Autodesk Fusion 360 part; units mm, degrees
(part 8 of 11)
  spline S18 degree 5 poles (-122.968, -126.8819) (-122.9875, -126.9008) (-123.0258, -126.9391) (-123.0815, -126.9984) (-123.1522, -127.0804) (-123.2358, -127.1873) (-123.3161, -127.2972) (-123.3942, -127.4089) (-123.4713, -127.5216) (-123.5476, -127.6349) (-123.623, -127.749) (-123.6973, -127.864) (-123.77, -127.9803) (-123.841, -128.098) (-123.9102, -128.2172) (-123.9778, -128.3376) (-124.0441, -128.459) (-124.1092, -128.5813) (-124.1732, -128.7044) (-124.2363, -128.8282) (-124.2984, -128.9527) (-124.3594, -129.078) (-124.4193, -129.2041) (-124.478, -129.3309) (-124.5356, -129.4586) (-124.5921, -129.5871) (-124.6476, -129.7162) (-124.7021, -129.846) (-124.7556, -129.9764) (-124.8082, -130.1075) (-124.8598, -130.2391) (-124.9105, -130.3714) (-124.9603, -130.5042) (-125.009, -130.6377) (-125.0569, -130.7717) (-125.1038, -130.9063) (-125.1498, -131.0414) (-125.1949, -131.1771) (-125.2391, -131.3133) (-125.2824, -131.45) (-125.3248, -131.5872) (-125.3664, -131.7249) (-125.4071, -131.8631) (-125.4469, -132.0017) (-125.4859, -132.1409) (-125.524, -132.2804) (-125.5613, -132.4205) (-125.5977, -132.561) (-125.6333, -132.7019) (-125.6681, -132.8432) (-125.702, -132.9849) (-125.7351, -133.1271) (-125.7674, -133.2697) (-125.7989, -133.4126) (-125.8295, -133.556) (-125.8594, -133.6997) (-125.8884, -133.8439) (-125.9167, -133.9883) (-125.9441, -134.1332) (-125.9708, -134.2784) (-125.9967, -134.424) (-126.0218, -134.5699) (-126.046, -134.7161) (-126.0696, -134.8627) (-126.0923, -135.0096) (-126.1143, -135.1569) (-126.1354, -135.3044) (-126.1559, -135.4523) (-126.1755, -135.6004) (-126.1944, -135.7489) (-126.2125, -135.8977) (-126.2264, -136.0169) (-126.2365, -136.1065) (-126.243, -136.1663) (-126.2463, -136.1962) knots 0 0 0 0 0 0 0.01428571 0.02857143 0.04285714 0.05714286 0.07142857 0.08571429 0.1 0.11428571 0.12857143 0.14285714 0.15714286 0.17142857 0.18571429 0.2 0.21428571 0.22857143 0.24285714 0.25714286 0.27142857 0.28571429 0.3 0.31428571 0.32857143 0.34285714 0.35714286 0.37142857 0.38571429 0.4 0.41428571 0.42857143 0.44285714 0.45714286 0.47142857 0.48571429 0.5 0.51428571 0.52857143 0.54285714 0.55714286 0.57142857 0.58571429 0.6 0.61428571 0.62857143 0.64285714 0.65714286 0.67142857 0.68571429 0.7 0.71428571 0.72857143 0.74285714 0.75714286 0.77142857 0.78571429 0.8 0.81428571 0.82857143 0.84285714 0.85714286 0.87142857 0.88571429 0.9 0.91428571 0.92857143 0.94285714 0.95714286 0.97142857 0.98571429 1 1 1 1 1 1
  arc A38 (-126.2463, -136.1962) -> (-123.0401, -138.7531) centre (-92.9957, -97.79) ccw
  spline S19 degree 5 poles (-123.0401, -138.7531) (-123.0117, -138.7432) (-122.9548, -138.7235) (-122.8698, -138.6938) (-122.7566, -138.6537) (-122.6156, -138.6029) (-122.475, -138.5515) (-122.3349, -138.4994) (-122.1953, -138.4465) (-122.0562, -138.3931) (-121.9175, -138.3389) (-121.7794, -138.284) (-121.6417, -138.2285) (-121.5045, -138.1723) (-121.3678, -138.1153) (-121.2317, -138.0577) (-121.096, -137.9994) (-120.9609, -137.9404) (-120.8264, -137.8807) (-120.6923, -137.8203) (-120.5588, -137.7593) (-120.4259, -137.6975) (-120.2935, -137.635) (-120.1617, -137.5718) (-120.0305, -137.5078) (-119.8998, -137.4432) (-119.7698, -137.3779) (-119.6403, -137.3118) (-119.5115, -137.2451) (-119.3832, -137.1776) (-119.2556, -137.1093) (-119.1287, -137.0404) (-119.0023, -136.9707) (-118.8767, -136.9003) (-118.7517, -136.8291) (-118.6274, -136.7572) (-118.5037, -136.6845) (-118.3808, -136.6111) (-118.2586, -136.537) (-118.137, -136.4621) (-118.0163, -136.3864) (-117.8962, -136.3099) (-117.777, -136.2327) (-117.6585, -136.1546) (-117.5409, -136.0758) (-117.424, -135.9962) (-117.308, -135.9157) (-117.1927, -135.8345) (-117.0783, -135.7525) (-116.9647, -135.6697) (-116.8521, -135.586) (-116.7404, -135.5014) (-116.6298, -135.4159) (-116.5202, -135.3295) (-116.4117, -135.2422) (-116.3041, -135.1539) (-116.1974, -135.0649) (-116.0917, -134.975) (-115.9869, -134.8844) (-115.8833, -134.7927) (-115.7809, -134.7) (-115.6802, -134.606) (-115.5812, -134.5107) (-115.484, -134.4139) (-115.3884, -134.3159) (-115.294, -134.217) (-115.2004, -134.1174) (-115.1077, -134.0172) (-115.0162, -133.9161) (-114.9269, -133.8134) (-114.8414, -133.7081) (-114.7771, -133.6209) (-114.7318, -133.5535) (-114.7029, -133.5075) (-114.6888, -133.4843) knots -1 -1 -1 -1 -1 -1 -0.98571429 -0.97142857 -0.95714286 -0.94285714 -0.92857143 -0.91428571 -0.9 -0.88571429 -0.87142857 -0.85714286 -0.84285714 -0.82857143 -0.81428571 -0.8 -0.78571429 -0.77142857 -0.75714286 -0.74285714 -0.72857143 -0.71428571 -0.7 -0.68571429 -0.67142857 -0.65714286 -0.64285714 -0.62857143 -0.61428571 -0.6 -0.58571429 -0.57142857 -0.55714286 -0.54285714 -0.52857143 -0.51428571 -0.5 -0.48571429 -0.47142857 -0.45714286 -0.44285714 -0.42857143 -0.41428571 -0.4 -0.38571429 -0.37142857 -0.35714286 -0.34285714 -0.32857143 -0.31428571 -0.3 -0.28571429 -0.27142857 -0.25714286 -0.24285714 -0.22857143 -0.21428571 -0.2 -0.18571429 -0.17142857 -0.15714286 -0.14285714 -0.12857143 -0.11428571 -0.1 -0.08571429 -0.07142857 -0.05714286 -0.04285714 -0.02857143 -0.01428571 0 0 0 0 0 0
  line L19 (-114.6888, -133.4843) -> (-112.5177, -129.913)
  arc A39 (-111.4416, -129.6385) -> (-112.5177, -129.913) centre (-111.8394, -130.3253) ccw
  arc A40 (-111.4416, -129.6385) -> (-106.395, -132.0688) centre (-92.9957, -97.79) ccw
  arc A41 (-105.9388, -133.0812) -> (-106.395, -132.0688) centre (-106.684, -132.808) ccw
  line L20 (-105.9388, -133.0812) -> (-107.3773, -137.0054)
  spline S20 degree 5 poles (-107.3773, -137.0054) (-107.3867, -137.0308) (-107.4046, -137.082) (-107.429, -137.1595) (-107.4571, -137.2642) (-107.4861, -137.3967) (-107.5107, -137.5305) (-107.5327, -137.6651) (-107.5532, -137.8001) (-107.5728, -137.9353) (-107.5912, -138.0708) (-107.6082, -138.2067) (-107.6233, -138.343) (-107.6361, -138.4799) (-107.6468, -138.6172) (-107.6555, -138.755) (-107.6625, -138.8932) (-107.6681, -139.0316) (-107.6724, -139.1703) (-107.6755, -139.3092) (-107.6774, -139.4483) (-107.678, -139.5877) (-107.6773, -139.7272) (-107.6751, -139.867) (-107.6716, -140.0071) (-107.6668, -140.1473) (-107.6608, -140.2877) (-107.6536, -140.4283) (-107.6452, -140.5691) (-107.6357, -140.71) (-107.6251, -140.851) (-107.6134, -140.9921) (-107.6006, -141.1334) (-107.5866, -141.2748) (-107.5716, -141.4163) (-107.5554, -141.5579) (-107.5383, -141.6996) (-107.52, -141.8414) (-107.5007, -141.9833) (-107.4805, -142.1253) (-107.4592, -142.2673) (-107.4369, -142.4094) (-107.4136, -142.5515) (-107.3893, -142.6937) (-107.3641, -142.836) (-107.3378, -142.9783) (-107.3107, -143.1206) (-107.2825, -143.263) (-107.2535, -143.4054) (-107.2235, -143.5478) (-107.1925, -143.6903) (-107.1607, -143.8327) (-107.1279, -143.9752) (-107.0942, -144.1176) (-107.0597, -144.2601) (-107.0242, -144.4026) (-106.9878, -144.545) (-106.9506, -144.6874) (-106.9125, -144.8299) (-106.8735, -144.9723) (-106.8336, -145.1146) (-106.7929, -145.257) (-106.7514, -145.3993) (-106.709, -145.5416) (-106.6657, -145.6838) (-106.6216, -145.826) (-106.5767, -145.9681) (-106.5309, -146.1102) (-106.4843, -146.2522) (-106.4369, -146.3942) (-106.3887, -146.5361) (-106.3495, -146.6495) (-106.3197, -146.7346) (-106.2996, -146.7913) (-106.2896, -146.8197) knots 0 0 0 0 0 0 0.01428571 0.02857143 0.04285714 0.05714286 0.07142857 0.08571429 0.1 0.11428571 0.12857143 0.14285714 0.15714286 0.17142857 0.18571429 0.2 0.21428571 0.22857143 0.24285714 0.25714286 0.27142857 0.28571429 0.3 0.31428571 0.32857143 0.34285714 0.35714286 0.37142857 0.38571429 0.4 0.41428571 0.42857143 0.44285714 0.45714286 0.47142857 0.48571429 0.5 0.51428571 0.52857143 0.54285714 0.55714286 0.57142857 0.58571429 0.6 0.61428571 0.62857143 0.64285714 0.65714286 0.67142857 0.68571429 0.7 0.71428571 0.72857143 0.74285714 0.75714286 0.77142857 0.78571429 0.8 0.81428571 0.82857143 0.84285714 0.85714286 0.87142857 0.88571429 0.9 0.91428571 0.92857143 0.94285714 0.95714286 0.97142857 0.98571429 1 1 1 1 1 1
  arc A42 (-106.2896, -146.8197) -> (-102.2915, -147.7322) centre (-92.9957, -97.79) ccw
  spline S21 degree 5 poles (-102.2915, -147.7322) (-102.2702, -147.711) (-102.2275, -147.6686) (-102.1638, -147.6049) (-102.0792, -147.5197) (-101.9742, -147.4128) (-101.8699, -147.3054) (-101.7663, -147.1977) (-101.6634, -147.0895) (-101.5613, -146.981) (-101.4599, -146.872) (-101.3592, -146.7626) (-101.2592, -146.6528) (-101.16, -146.5426) (-101.0616, -146.4321) (-100.9639, -146.3211) (-100.867, -146.2097) (-100.7709, -146.0979) (-100.6755, -145.9858) (-100.581, -145.8732) (-100.4872, -145.7602) (-100.3942, -145.6469) (-100.3021, -145.5331) (-100.2107, -145.419) (-100.1202, -145.3045) (-100.0306, -145.1896) (-99.9417, -145.0743) (-99.8538, -144.9586) (-99.7666, -144.8425) (-99.6804, -144.7261) (-99.595, -144.6092) (-99.5106, -144.492) (-99.427, -144.3744) (-99.3443, -144.2565) (-99.2626, -144.1381) (-99.1818, -144.0194) (-99.1019, -143.9003) (-99.023, -143.7808) (-98.945, -143.661) (-98.8681, -143.5407) (-98.7921, -143.4202) (-98.7171, -143.2992) (-98.6432, -143.1778) (-98.5703, -143.0561) (-98.4985, -142.9341) (-98.4278, -142.8116) (-98.3581, -142.6888) (-98.2895, -142.5656) (-98.222, -142.4421) (-98.1557, -142.3182) (-98.0905, -142.1939) (-98.0266, -142.0693) (-97.964, -141.9442) (-97.9028, -141.8188) (-97.8428, -141.693) (-97.7842, -141.5669) (-97.7268, -141.4404) (-97.6705, -141.3135) (-97.6154, -141.1864) (-97.5618, -141.0589) (-97.5098, -140.9309) (-97.4598, -140.8025) (-97.412, -140.6737) (-97.3665, -140.5443) (-97.3228, -140.4145) (-97.2807, -140.2844) (-97.2396, -140.1541) (-97.1996, -140.0236) (-97.161, -139.8928) (-97.1251, -139.7616) (-97.0937, -139.6296) (-97.0736, -139.5231) (-97.062, -139.4427) (-97.0559, -139.3888) (-97.0533, -139.3617) knots -1 -1 -1 -1 -1 -1 -0.98571429 -0.97142857 -0.95714286 -0.94285714 -0.92857143 -0.91428571 -0.9 -0.88571429 -0.87142857 -0.85714286 -0.84285714 -0.82857143 -0.81428571 -0.8 -0.78571429 -0.77142857 -0.75714286 -0.74285714 -0.72857143 -0.71428571 -0.7 -0.68571429 -0.67142857 -0.65714286 -0.64285714 -0.62857143 -0.61428571 -0.6 -0.58571429 -0.57142857 -0.55714286 -0.54285714 -0.52857143 -0.51428571 -0.5 -0.48571429 -0.47142857 -0.45714286 -0.44285714 -0.42857143 -0.41428571 -0.4 -0.38571429 -0.37142857 -0.35714286 -0.34285714 -0.32857143 -0.31428571 -0.3 -0.28571429 -0.27142857 -0.25714286 -0.24285714 -0.22857143 -0.21428571 -0.2 -0.18571429 -0.17142857 -0.15714286 -0.14285714 -0.12857143 -0.11428571 -0.1 -0.08571429 -0.07142857 -0.05714286 -0.04285714 -0.02857143 -0.01428571 0 0 0 0 0 0
  line L21 (-97.0533, -139.3617) -> (-96.6467, -135.2021)
  arc A43 (-95.7964, -134.4878) -> (-96.6467, -135.2021) centre (-95.8568, -135.2793) ccw
  arc A44 (-95.7964, -134.4878) -> (-90.1951, -134.4878) centre (-92.9957, -97.79) ccw
  arc A45 (-89.3447, -135.2021) -> (-90.1951, -134.4878) centre (-90.1347, -135.2793) ccw
  line L22 (-89.3447, -135.2021) -> (-88.9382, -139.3617)
  spline S22 degree 5 poles (-88.9382, -139.3617) (-88.9355, -139.3888) (-88.9294, -139.4427) (-88.9178, -139.5231) (-88.8978, -139.6296) (-88.8664, -139.7616) (-88.8305, -139.8928) (-88.7919, -140.0236) (-88.7518, -140.1541) (-88.7108, -140.2844) (-88.6686, -140.4145) (-88.625, -140.5443) (-88.5794, -140.6737) (-88.5316, -140.8025) (-88.4816, -140.9309) (-88.4297, -141.0589) (-88.376, -141.1864) (-88.321, -141.3135) (-88.2647, -141.4404) (-88.2072, -141.5669) (-88.1486, -141.693) (-88.0887, -141.8188) (-88.0274, -141.9442) (-87.9649, -142.0693) (-87.9009, -142.1939) (-87.8358, -142.3182) (-87.7694, -142.4421) (-87.7019, -142.5656) (-87.6333, -142.6888) (-87.5636, -142.8116) (-87.4929, -142.9341) (-87.4211, -143.0561) (-87.3482, -143.1778) (-87.2743, -143.2992) (-87.1994, -143.4202) (-87.1234, -143.5407) (-87.0464, -143.661) (-86.9684, -143.7808) (-86.8895, -143.9003) (-86.8097, -144.0194) (-86.7288, -144.1381) (-86.6471, -144.2565) (-86.5645, -144.3744) (-86.4809, -144.492) (-86.3964, -144.6092) (-86.311, -144.7261) (-86.2248, -144.8425) (-86.1377, -144.9586) (-86.0497, -145.0743) (-85.9609, -145.1896) (-85.8712, -145.3045) (-85.7807, -145.419) (-85.6894, -145.5331) (-85.5972, -145.6469) (-85.5042, -145.7602) (-85.4105, -145.8732) (-85.3159, -145.9858) (-85.2206, -146.0979) (-85.1244, -146.2097) (-85.0275, -146.3211) (-84.9299, -146.4321) (-84.8314, -146.5426) (-84.7322, -146.6528) (-84.6323, -146.7626) (-84.5316, -146.872) (-84.4302, -146.981) (-84.328, -147.0895) (-84.2251, -147.1977) (-84.1215, -147.3054) (-84.0172, -147.4128) (-83.9122, -147.5197) (-83.8276, -147.6049) (-83.7639, -147.6686) (-83.7212, -147.711) (-83.6999, -147.7322) knots 0 0 0 0 0 0 0.01428571 0.02857143 0.04285714 0.05714286 0.07142857 0.08571429 0.1 0.11428571 0.12857143 0.14285714 0.15714286 0.17142857 0.18571429 0.2 0.21428571 0.22857143 0.24285714 0.25714286 0.27142857 0.28571429 0.3 0.31428571 0.32857143 0.34285714 0.35714286 0.37142857 0.38571429 0.4 0.41428571 0.42857143 0.44285714 0.45714286 0.47142857 0.48571429 0.5 0.51428571 0.52857143 0.54285714 0.55714286 0.57142857 0.58571429 0.6 0.61428571 0.62857143 0.64285714 0.65714286 0.67142857 0.68571429 0.7 0.71428571 0.72857143 0.74285714 0.75714286 0.77142857 0.78571429 0.8 0.81428571 0.82857143 0.84285714 0.85714286 0.87142857 0.88571429 0.9 0.91428571 0.92857143 0.94285714 0.95714286 0.97142857 0.98571429 1 1 1 1 1 1
  arc A46 (-83.6999, -147.7322) -> (-79.7018, -146.8197) centre (-92.9957, -97.79) ccw
  spline S23 degree 5 poles (-79.7018, -146.8197) (-79.6918, -146.7913) (-79.6718, -146.7346) (-79.642, -146.6495) (-79.6027, -146.5361) (-79.5545, -146.3942) (-79.5071, -146.2522) (-79.4605, -146.1102) (-79.4148, -145.9681) (-79.3698, -145.826) (-79.3257, -145.6838) (-79.2825, -145.5416) (-79.2401, -145.3993) (-79.1985, -145.257) (-79.1578, -145.1146) (-79.1179, -144.9723) (-79.079, -144.8299) (-79.0408, -144.6874) (-79.0036, -144.545) (-78.9672, -144.4026) (-78.9318, -144.2601) (-78.8972, -144.1176) (-78.8635, -143.9752) (-78.8308, -143.8327) (-78.7989, -143.6903) (-78.768, -143.5478) (-78.738, -143.4054) (-78.7089, -143.263) (-78.6808, -143.1206) (-78.6536, -142.9783) (-78.6274, -142.836) (-78.6021, -142.6937) (-78.5778, -142.5515) (-78.5546, -142.4094) (-78.5323, -142.2673) (-78.511, -142.1253) (-78.4907, -141.9833) (-78.4714, -141.8414) (-78.4532, -141.6996) (-78.436, -141.5579) (-78.4199, -141.4163) (-78.4048, -141.2748) (-78.3908, -141.1334) (-78.378, -140.9921) (-78.3663, -140.851) (-78.3557, -140.71) (-78.3462, -140.5691) (-78.3379, -140.4283) (-78.3306, -140.2877) (-78.3246, -140.1473) (-78.3198, -140.0071) (-78.3163, -139.867) (-78.3142, -139.7272) (-78.3134, -139.5877) (-78.314, -139.4483) (-78.3159, -139.3092) (-78.319, -139.1703) (-78.3234, -139.0316) (-78.3289, -138.8932) (-78.3359, -138.755) (-78.3446, -138.6172) (-78.3553, -138.4799) (-78.3681, -138.343) (-78.3832, -138.2067) (-78.4002, -138.0708) (-78.4187, -137.9353) (-78.4382, -137.8001) (-78.4588, -137.6651) (-78.4807, -137.5305) (-78.5053, -137.3967) (-78.5343, -137.2642) (-78.5624, -137.1595) (-78.5869, -137.082) (-78.6048, -137.0308) (-78.6141, -137.0054) knots -1 -1 -1 -1 -1 -1 -0.98571429 -0.97142857 -0.95714286 -0.94285714 -0.92857143 -0.91428571 -0.9 -0.88571429 -0.87142857 -0.85714286 -0.84285714 -0.82857143 -0.81428571 -0.8 -0.78571429 -0.77142857 -0.75714286 -0.74285714 -0.72857143 -0.71428571 -0.7 -0.68571429 -0.67142857 -0.65714286 -0.64285714 -0.62857143 -0.61428571 -0.6 -0.58571429 -0.57142857 -0.55714286 -0.54285714 -0.52857143 -0.51428571 -0.5 -0.48571429 -0.47142857 -0.45714286 -0.44285714 -0.42857143 -0.41428571 -0.4 -0.38571429 -0.37142857 -0.35714286 -0.34285714 -0.32857143 -0.31428571 -0.3 -0.28571429 -0.27142857 -0.25714286 -0.24285714 -0.22857143 -0.21428571 -0.2 -0.18571429 -0.17142857 -0.15714286 -0.14285714 -0.12857143 -0.11428571 -0.1 -0.08571429 -0.07142857 -0.05714286 -0.04285714 -0.02857143 -0.01428571 0 0 0 0 0 0
  line L23 (-78.6141, -137.0054) -> (-80.0527, -133.0812)
  arc A47 (-79.5964, -132.0688) -> (-80.0527, -133.0812) centre (-79.3074, -132.808) ccw
  arc A48 (-79.5964, -132.0688) -> (-74.5498, -129.6385) centre (-92.9957, -97.79) ccw
  arc A49 (-73.4737, -129.913) -> (-74.5498, -129.6385) centre (-74.152, -130.3253) ccw
  line L24 (-73.4737, -129.913) -> (-71.3027, -133.4843)
  spline S24 degree 5 poles (-71.3027, -133.4843) (-71.2886, -133.5075) (-71.2597, -133.5535) (-71.2143, -133.6209) (-71.1501, -133.7081) (-71.0645, -133.8134) (-70.9752, -133.9161) (-70.8837, -134.0172) (-70.791, -134.1174) (-70.6974, -134.217) (-70.603, -134.3159) (-70.5074, -134.4139) (-70.4102, -134.5107) (-70.3112, -134.606) (-70.2105, -134.7) (-70.1082, -134.7927) (-70.0045, -134.8844) (-69.8997, -134.975) (-69.794, -135.0649) (-69.6874, -135.1539) (-69.5798, -135.2422) (-69.4712, -135.3295) (-69.3616, -135.4159) (-69.251, -135.5014) (-69.1393, -135.586) (-69.0267, -135.6697) (-68.9131, -135.7525) (-68.7987, -135.8345) (-68.6835, -135.9157) (-68.5674, -135.9962) (-68.4506, -136.0758) (-68.3329, -136.1546) (-68.2145, -136.2327) (-68.0952, -136.3099) (-67.9752, -136.3864) (-67.8544, -136.4621) (-67.7329, -136.537) (-67.6106, -136.6111) (-67.4877, -136.6845) (-67.3641, -136.7572) (-67.2398, -136.8291) (-67.1148, -136.9003) (-66.9891, -136.9707) (-66.8628, -137.0404) (-66.7358, -137.1093) (-66.6082, -137.1776) (-66.48, -137.2451) (-66.3511, -137.3118) (-66.2217, -137.3779) (-66.0916, -137.4432) (-65.961, -137.5078) (-65.8297, -137.5718) (-65.6979, -137.635) (-65.5656, -137.6975) (-65.4326, -137.7593) (-65.2991, -137.8203) (-65.1651, -137.8807) (-65.0305, -137.9404) (-64.8954, -137.9994) (-64.7598, -138.0577) (-64.6236, -138.1153) (-64.4869, -138.1723) (-64.3498, -138.2285) (-64.2121, -138.284) (-64.0739, -138.3389) (-63.9352, -138.3931) (-63.7961, -138.4465) (-63.6565, -138.4994) (-63.5164, -138.5515) (-63.3759, -138.6029) (-63.2349, -138.6537) (-63.1217, -138.6938) (-63.0366, -138.7235) (-62.9798, -138.7432) (-62.9513, -138.7531) knots 0 0 0 0 0 0 0.01428571 0.02857143 0.04285714 0.05714286 0.07142857 0.08571429 0.1 0.11428571 0.12857143 0.14285714 0.15714286 0.17142857 0.18571429 0.2 0.21428571 0.22857143 0.24285714 0.25714286 0.27142857 0.28571429 0.3 0.31428571 0.32857143 0.34285714 0.35714286 0.37142857 0.38571429 0.4 0.41428571 0.42857143 0.44285714 0.45714286 0.47142857 0.48571429 0.5 0.51428571 0.52857143 0.54285714 0.55714286 0.57142857 0.58571429 0.6 0.61428571 0.62857143 0.64285714 0.65714286 0.67142857 0.68571429 0.7 0.71428571 0.72857143 0.74285714 0.75714286 0.77142857 0.78571429 0.8 0.81428571 0.82857143 0.84285714 0.85714286 0.87142857 0.88571429 0.9 0.91428571 0.92857143 0.94285714 0.95714286 0.97142857 0.98571429 1 1 1 1 1 1
  arc A50 (-62.9513, -138.7531) -> (-59.7452, -136.1962) centre (-92.9957, -97.79) ccw
  spline S25 degree 5 poles (-59.7452, -136.1962) (-59.7484, -136.1663) (-59.755, -136.1065) (-59.765, -136.0169) (-59.7789, -135.8977) (-59.797, -135.7489) (-59.8159, -135.6004) (-59.8356, -135.4523) (-59.856, -135.3044) (-59.8772, -135.1569) (-59.8991, -135.0096) (-59.9219, -134.8627) (-59.9454, -134.7161) (-59.9697, -134.5699) (-59.9948, -134.424) (-60.0206, -134.2784) (-60.0473, -134.1332) (-60.0747, -133.9883) (-60.103, -133.8439) (-60.132, -133.6997) (-60.1619, -133.556) (-60.1926, -133.4126) (-60.224, -133.2697) (-60.2563, -133.1271) (-60.2894, -132.9849) (-60.3234, -132.8432) (-60.3581, -132.7019) (-60.3937, -132.561) (-60.4302, -132.4205) (-60.4674, -132.2804) (-60.5055, -132.1409) (-60.5445, -132.0017) (-60.5843, -131.8631) (-60.625, -131.7249) (-60.6666, -131.5872) (-60.709, -131.45) (-60.7524, -131.3133) (-60.7966, -131.1771) (-60.8417, -131.0414) (-60.8877, -130.9063) (-60.9346, -130.7717) (-60.9824, -130.6377) (-61.0312, -130.5042) (-61.0809, -130.3714) (-61.1316, -130.2391) (-61.1832, -130.1075) (-61.2358, -129.9764) (-61.2893, -129.846) (-61.3438, -129.7162) (-61.3993, -129.5871) (-61.4558, -129.4586) (-61.5135, -129.3309) (-61.5722, -129.2041) (-61.6321, -129.078) (-61.6931, -128.9527) (-61.7551, -128.8282) (-61.8182, -128.7044) (-61.8823, -128.5813) (-61.9474, -128.459) (-62.0136, -128.3376) (-62.0812, -128.2172) (-62.1505, -128.098) (-62.2214, -127.9803) (-62.2941, -127.864) (-62.3684, -127.749) (-62.4438, -127.6349) (-62.5201, -127.5216) (-62.5972, -127.4089) (-62.6754, -127.2972) (-62.7556, -127.1873) (-62.8392, -127.0804) (-62.9099, -126.9984) (-62.9656, -126.9391) (-63.0039, -126.9008) (-63.0234, -126.8819) knots -1 -1 -1 -1 -1 -1 -0.98571429 -0.97142857 -0.95714286 -0.94285714 -0.92857143 -0.91428571 -0.9 -0.88571429 -0.87142857 -0.85714286 -0.84285714 -0.82857143 -0.81428571 -0.8 -0.78571429 -0.77142857 -0.75714286 -0.74285714 -0.72857143 -0.71428571 -0.7 -0.68571429 -0.67142857 -0.65714286 -0.64285714 -0.62857143 -0.61428571 -0.6 -0.58571429 -0.57142857 -0.55714286 -0.54285714 -0.52857143 -0.51428571 -0.5 -0.48571429 -0.47142857 -0.45714286 -0.44285714 -0.42857143 -0.41428571 -0.4 -0.38571429 -0.37142857 -0.35714286 -0.34285714 -0.32857143 -0.31428571 -0.3 -0.28571429 -0.27142857 -0.25714286 -0.24285714 -0.22857143 -0.21428571 -0.2 -0.18571429 -0.17142857 -0.15714286 -0.14285714 -0.12857143 -0.11428571 -0.1 -0.08571429 -0.07142857 -0.05714286 -0.04285714 -0.02857143 -0.01428571 0 0 0 0 0 0
  line L25 (-63.0234, -126.8819) -> (-66.0221, -123.9705)
  arc A51 (-66.0503, -122.8603) -> (-66.0221, -123.9705) centre (-65.4692, -123.401) ccw
  arc A52 (-66.0503, -122.8603) -> (-62.558, -118.4811) centre (-92.9957, -97.79) ccw
  arc A53 (-61.4694, -118.2616) -> (-62.558, -118.4811) centre (-61.9015, -118.9273) ccw
  line L26 (-61.4694, -118.2616) -> (-57.9637, -120.5372)
  spline S26 degree 5 poles (-57.9637, -120.5372) (-57.941, -120.552) (-57.895, -120.5808) (-57.8249, -120.6219) (-57.7292, -120.6726) (-57.6064, -120.7304) (-57.4814, -120.7841) (-57.3551, -120.8355) (-57.2281, -120.8856) (-57.1006, -120.9347) (-56.9726, -120.9829) (-56.8439, -121.0297) (-56.7144, -121.0747) (-56.5838, -121.1177) (-56.4523, -121.1587) (-56.3198, -121.1978) (-56.1867, -121.2354) (-56.053, -121.2716) (-55.9187, -121.3067) (-55.784, -121.3406) (-55.6488, -121.3734) (-55.5131, -121.405) (-55.3768, -121.4353) (-55.2401, -121.4644) (-55.1028, -121.4921) (-54.965, -121.5186) (-54.8267, -121.544) (-54.6881, -121.5682) (-54.549, -121.5914) (-54.4095, -121.6135) (-54.2697, -121.6346) (-54.1295, -121.6546) (-53.9889, -121.6735) (-53.8479, -121.6913) (-53.7066, -121.7081) (-53.565, -121.7239) (-53.423, -121.7387) (-53.2807, -121.7525) (-53.1381, -121.7653) (-52.9951, -121.7771) (-52.8519, -121.7879) (-52.7085, -121.7978) (-52.5647, -121.8067) (-52.4206, -121.8147) (-52.2763, -121.8217) (-52.1318, -121.8278) (-51.9869, -121.833) (-51.8419, -121.8373) (-51.6966, -121.8406) (-51.5511, -121.8431) (-51.4053, -121.8446) (-51.2593, -121.8452) (-51.1132, -121.845) (-50.9668, -121.8439) (-50.8202, -121.8419) (-50.6734, -121.839) (-50.5264, -121.8352) (-50.3793, -121.8306) (-50.232, -121.8252) (-50.0845, -121.8188) (-49.9368, -121.8117) (-49.789, -121.8037) (-49.641, -121.7948) (-49.4928, -121.7851) (-49.3445, -121.7746) (-49.1961, -121.7632) (-49.0475, -121.751) (-48.8988, -121.738) (-48.75, -121.7242) (-48.6011, -121.7096) (-48.452, -121.6942) (-48.3326, -121.6812) (-48.2431, -121.6711) (-48.1833, -121.6642) (-48.1534, -121.6607) knots 0 0 0 0 0 0 0.01428571 0.02857143 0.04285714 0.05714286 0.07142857 0.08571429 0.1 0.11428571 0.12857143 0.14285714 0.15714286 0.17142857 0.18571429 0.2 0.21428571 0.22857143 0.24285714 0.25714286 0.27142857 0.28571429 0.3 0.31428571 0.32857143 0.34285714 0.35714286 0.37142857 0.38571429 0.4 0.41428571 0.42857143 0.44285714 0.45714286 0.47142857 0.48571429 0.5 0.51428571 0.52857143 0.54285714 0.55714286 0.57142857 0.58571429 0.6 0.61428571 0.62857143 0.64285714 0.65714286 0.67142857 0.68571429 0.7 0.71428571 0.72857143 0.74285714 0.75714286 0.77142857 0.78571429 0.8 0.81428571 0.82857143 0.84285714 0.85714286 0.87142857 0.88571429 0.9 0.91428571 0.92857143 0.94285714 0.95714286 0.97142857 0.98571429 1 1 1 1 1 1
  arc A54 (-48.1534, -121.6607) -> (-46.3741, -117.9659) centre (-92.9957, -97.79) ccw
  spline S27 degree 5 poles (-46.3741, -117.9659) (-46.39, -117.9404) (-46.4219, -117.8894) (-46.4698, -117.813) (-46.5341, -117.7116) (-46.615, -117.5854) (-46.6964, -117.4599) (-46.7784, -117.3349) (-46.8609, -117.2105) (-46.9441, -117.0868) (-47.0277, -116.9637) (-47.112, -116.8412) (-47.1967, -116.7193) (-47.2821, -116.5981) (-47.368, -116.4775) (-47.4545, -116.3576) (-47.5415, -116.2383) (-47.6291, -116.1197) (-47.7172, -116.0018) (-47.8059, -115.8845) (-47.8952, -115.768) (-47.985, -115.6521) (-48.0754, -115.537) (-48.1663, -115.4225) (-48.2578, -115.3088) (-48.3499, -115.1958) (-48.4426, -115.0836) (-48.5358, -114.9721) (-48.6295, -114.8613) (-48.7239, -114.7513) (-48.8188, -114.6421) (-48.9143, -114.5336) (-49.0103, -114.426) (-49.1069, -114.3192) (-49.2041, -114.2131) (-49.3019, -114.1079) (-49.4002, -114.0036) (-49.4991, -113.9) (-49.5986, -113.7974) (-49.6987, -113.6956) (-49.7994, -113.5947) (-49.9006, -113.4947) (-50.0025, -113.3956) (-50.1049, -113.2975) (-50.208, -113.2003) (-50.3116, -113.1041) (-50.4158, -113.0089) (-50.5207, -112.9146) (-50.6261, -112.8213) (-50.7321, -112.729) (-50.8388, -112.6378) (-50.9461, -112.5478) (-51.054, -112.4589) (-51.1627, -112.3713) (-51.272, -112.2849) (-51.3819, -112.1997) (-51.4925, -112.1155) (-51.6036, -112.0324) (-51.7153, -111.9504) (-51.8277, -111.8698) (-51.9409, -111.7906) (-52.0549, -111.7133) (-52.1699, -111.6381) (-52.2859, -111.5649) (-52.4027, -111.4934) (-52.5202, -111.4234) (-52.6381, -111.3544) (-52.7564, -111.2863) (-52.8753, -111.2195) (-52.9953, -111.1553) (-53.117, -111.0954) (-53.2163, -111.0521) (-53.2922, -111.0229) (-53.3434, -111.005) (-53.3691, -110.9964) knots -1 -1 -1 -1 -1 -1 -0.98571429 -0.97142857 -0.95714286 -0.94285714 -0.92857143 -0.91428571 -0.9 -0.88571429 -0.87142857 -0.85714286 -0.84285714 -0.82857143 -0.81428571 -0.8 -0.78571429 -0.77142857 -0.75714286 -0.74285714 -0.72857143 -0.71428571 -0.7 -0.68571429 -0.67142857 -0.65714286 -0.64285714 -0.62857143 -0.61428571 -0.6 -0.58571429 -0.57142857 -0.55714286 -0.54285714 -0.52857143 -0.51428571 -0.5 -0.48571429 -0.47142857 -0.45714286 -0.44285714 -0.42857143 -0.41428571 -0.4 -0.38571429 -0.37142857 -0.35714286 -0.34285714 -0.32857143 -0.31428571 -0.3 -0.28571429 -0.27142857 -0.25714286 -0.24285714 -0.22857143 -0.21428571 -0.2 -0.18571429 -0.17142857 -0.15714286 -0.14285714 -0.12857143 -0.11428571 -0.1 -0.08571429 -0.07142857 -0.05714286 -0.04285714 -0.02857143 -0.01428571 0 0 0 0 0 0
  line L27 (-53.3691, -110.9964) -> (-57.334, -109.6744)
  arc A55 (-57.8411, -108.6864) -> (-57.334, -109.6744) centre (-57.083, -108.9214) ccw
  circle A56 centre (-92.9957, -97.79) radius 5
  circle A57 centre (-92.9957, -97.79) radius 10 construction
  line L28 (-102.9957, -87.79) -> (-82.9957, -87.79)
  line L29 (-82.9957, -87.79) -> (-82.9957, -107.79)
  line L30 (-82.9957, -107.79) -> (-102.9957, -107.79)
  line L31 (-102.9957, -107.79) -> (-102.9957, -87.79)
  dimension "d112" = 5
  dimension "d113" = 20
  dimension "d114" = 20
  constraint horizontal L28
  constraint vertical L29
  constraint horizontal L30
  constraint vertical L31
  constraint tangent A57 L28
  constraint tangent A57 L29
  measures "d112" distance of A56
  measures "d113" distance of L28.start L28.end
  measures "d114" distance of L28.end L29.end
extrude "Extrude3'" add sketch "Sketch4" along normal blind 20 contours L28 L29 L30 L31 sketch seen with x (1, 0, 0) y (0, 1, 0) z (0, 0, 1) at (12.0054, 91.2413, 0) bodies 2 in component "Spur Gear (14 teeth)"
sketch "Sketch5" plane through (0, 0, 12.5) normal (0, 0, -1) x (-1, 0, 0)
  circle A0 centre (-50, -10) radius 2.75
  circle A1 centre (50, 10) radius 2.75
  circle A2 centre (-50, 10) radius 2.75
  circle A3 centre (50, -10) radius 2.75
  circle A4 centre (0.5538, 0.6546) radius 15.5
  arc A5 (-75.7049, -29.609) -> (-75.2572, -28.5856) centre (-75.9978, -28.8713) ccw
  line L0 (-75.7049, -29.609) -> (-77.0937, -30.1604)
  spline S0 degree 5 poles (-77.0937, -30.1604) (-77.1259, -30.1732) (-77.1899, -30.1995) (-77.2849, -30.2412) (-77.4095, -30.3012) (-77.5625, -30.3821) (-77.7135, -30.4672) (-77.8634, -30.5549) (-78.0125, -30.644) (-78.1613, -30.7341) (-78.3095, -30.8251) (-78.4571, -30.9174) (-78.6037, -31.0115) (-78.7494, -31.1075) (-78.894, -31.2056) (-79.0377, -31.3055) (-79.1805, -31.407) (-79.3226, -31.5098) (-79.4641, -31.6138) (-79.605, -31.7187) (-79.7453, -31.8248) (-79.885, -31.9319) (-80.024, -32.0402) (-80.1623, -32.1498) (-80.2999, -32.2605) (-80.4368, -32.3724) (-80.5731, -32.4853) (-80.7088, -32.5993) (-80.8439, -32.7142) (-80.9784, -32.8301) (-81.1124, -32.9469) (-81.2457, -33.0647) (-81.3785, -33.1834) (-81.5106, -33.303) (-81.6422, -33.4236) (-81.7732, -33.545) (-81.9037, -33.6674) (-82.0336, -33.7906) (-82.1629, -33.9146) (-82.2917, -34.0395) (-82.4199, -34.1651) (-82.5476, -34.2916) (-82.6747, -34.4189) (-82.8013, -34.547) (-82.9273, -34.6759) (-83.0528, -34.8055) (-83.1778, -34.936) (-83.3022, -35.0671) (-83.4261, -35.199) (-83.5495, -35.3317) (-83.6723, -35.4651) (-83.7947, -35.5992) (-83.9165, -35.734) (-84.0377, -35.8695) (-84.1585, -36.0057) (-84.2787, -36.1426) (-84.3985, -36.2802) (-84.5177, -36.4185) (-84.6364, -36.5574) (-84.7546, -36.697) (-84.8723, -36.8372) (-84.9894, -36.9781) (-85.1061, -37.1197) (-85.2222, -37.2619) (-85.3379, -37.4047) (-85.453, -37.5482) (-85.5677, -37.6922) (-85.6818, -37.8369) (-85.7955, -37.9822) (-85.9086, -38.1281) (-86.0212, -38.2746) (-86.111, -38.3923) (-86.178, -38.4808) (-86.2226, -38.54) (-86.2449, -38.5696) knots 0 0 0 0 0 0 0.01428571 0.02857143 0.04285714 0.05714286 0.07142857 0.08571429 0.1 0.11428571 0.12857143 0.14285714 0.15714286 0.17142857 0.18571429 0.2 0.21428571 0.22857143 0.24285714 0.25714286 0.27142857 0.28571429 0.3 0.31428571 0.32857143 0.34285714 0.35714286 0.37142857 0.38571429 0.4 0.41428571 0.42857143 0.44285714 0.45714286 0.47142857 0.48571429 0.5 0.51428571 0.52857143 0.54285714 0.55714286 0.57142857 0.58571429 0.6 0.61428571 0.62857143 0.64285714 0.65714286 0.67142857 0.68571429 0.7 0.71428571 0.72857143 0.74285714 0.75714286 0.77142857 0.78571429 0.8 0.81428571 0.82857143 0.84285714 0.85714286 0.87142857 0.88571429 0.9 0.91428571 0.92857143 0.94285714 0.95714286 0.97142857 0.98571429 1 1 1 1 1 1
  arc A6 (-86.2449, -38.5696) -> (-84.231, -42.7515) centre (0.5538, 0.6546) ccw
  spline S1 degree 5 poles (-71.9508, -40.8398) (-71.9808, -40.857) (-72.0413, -40.8906) (-72.1332, -40.9389) (-72.2578, -40.9989) (-72.4164, -41.0681) (-72.5771, -41.1331) (-72.7391, -41.1956) (-72.9018, -41.2566) (-73.0649, -41.3168) (-73.2285, -41.3759) (-73.3927, -41.4337) (-73.5577, -41.4898) (-73.7236, -41.5437) (-73.8904, -41.5957) (-74.0581, -41.6457) (-74.2265, -41.6941) (-74.3955, -41.7411) (-74.565, -41.7869) (-74.7349, -41.8316) (-74.9053, -41.8752) (-75.0761, -41.9176) (-75.2475, -41.9587) (-75.4193, -41.9985) (-75.5917, -42.0371) (-75.7646, -42.0744) (-75.9378, -42.1105) (-76.1116, -42.1456) (-76.2856, -42.1795) (-76.4601, -42.2125) (-76.635, -42.2443) (-76.8102, -42.2752) (-76.9858, -42.305) (-77.1617, -42.3337) (-77.338, -42.3614) (-77.5146, -42.3881) (-77.6916, -42.4138) (-77.8689, -42.4386) (-78.0465, -42.4623) (-78.2244, -42.4852) (-78.4026, -42.5071) (-78.5811, -42.528) (-78.7599, -42.548) (-78.939, -42.5671) (-79.1183, -42.5853) (-79.2979, -42.6026) (-79.4778, -42.619) (-79.658, -42.6345) (-79.8383, -42.6491) (-80.019, -42.6629) (-80.1998, -42.6758) (-80.381, -42.6878) (-80.5623, -42.699) (-80.7439, -42.7093) (-80.9257, -42.7188) (-81.1077, -42.7274) (-81.2899, -42.7353) (-81.4723, -42.7423) (-81.6549, -42.7484) (-81.8378, -42.7538) (-82.0208, -42.7584) (-82.204, -42.7621) (-82.3874, -42.7651) (-82.571, -42.7672) (-82.7548, -42.7686) (-82.9387, -42.7692) (-83.1228, -42.769) (-83.3071, -42.768) (-83.4916, -42.7663) (-83.6762, -42.7638) (-83.861, -42.7605) (-84.0089, -42.7573) (-84.1199, -42.7545) (-84.194, -42.7525) (-84.231, -42.7515) knots 0 0 0 0 0 0 0.01428571 0.02857143 0.04285714 0.05714286 0.07142857 0.08571429 0.1 0.11428571 0.12857143 0.14285714 0.15714286 0.17142857 0.18571429 0.2 0.21428571 0.22857143 0.24285714 0.25714286 0.27142857 0.28571429 0.3 0.31428571 0.32857143 0.34285714 0.35714286 0.37142857 0.38571429 0.4 0.41428571 0.42857143 0.44285714 0.45714286 0.47142857 0.48571429 0.5 0.51428571 0.52857143 0.54285714 0.55714286 0.57142857 0.58571429 0.6 0.61428571 0.62857143 0.64285714 0.65714286 0.67142857 0.68571429 0.7 0.71428571 0.72857143 0.74285714 0.75714286 0.77142857 0.78571429 0.8 0.81428571 0.82857143 0.84285714 0.85714286 0.87142857 0.88571429 0.9 0.91428571 0.92857143 0.94285714 0.95714286 0.97142857 0.98571429 1 1 1 1 1 1
  line L1 (-71.9508, -40.8398) -> (-70.6538, -40.0978)
  arc A7 (-69.5745, -40.3858) -> (-70.6538, -40.0978) centre (-70.2596, -40.7867) ccw
  arc A8 (-69.5745, -40.3858) -> (-66.8499, -44.7221) centre (0.5538, 0.6546) ccw
  arc A9 (-67.0586, -45.8194) -> (-66.8499, -44.7221) centre (-67.5084, -45.1653) ccw
  line L2 (-67.0586, -45.8194) -> (-68.2899, -46.666)
  spline S2 degree 5 poles (-68.2899, -46.666) (-68.3185, -46.6856) (-68.375, -46.7255) (-68.4583, -46.7874) (-68.5664, -46.8736) (-68.6976, -46.9865) (-68.826, -47.103) (-68.9525, -47.2219) (-69.0781, -47.342) (-69.2031, -47.4628) (-69.3273, -47.5846) (-69.4506, -47.7074) (-69.5727, -47.8317) (-69.6933, -47.9578) (-69.8125, -48.0856) (-69.9303, -48.215) (-70.047, -48.3457) (-70.1627, -48.4776) (-70.2775, -48.6104) (-70.3915, -48.7441) (-70.5047, -48.8787) (-70.617, -49.0142) (-70.7284, -49.1508) (-70.8389, -49.2883) (-70.9484, -49.4269) (-71.057, -49.5664) (-71.1647, -49.7069) (-71.2717, -49.8482) (-71.3778, -49.9903) (-71.4832, -50.1332) (-71.5878, -50.2769) (-71.6916, -50.4214) (-71.7946, -50.5667) (-71.8968, -50.7127) (-71.9983, -50.8595) (-72.099, -51.0071) (-72.1989, -51.1554) (-72.2982, -51.3044) (-72.3966, -51.4541) (-72.4944, -51.6045) (-72.5914, -51.7555) (-72.6878, -51.9073) (-72.7834, -52.0596) (-72.8783, -52.2127) (-72.9725, -52.3664) (-73.066, -52.5207) (-73.1588, -52.6757) (-73.2509, -52.8312) (-73.3424, -52.9874) (-73.4331, -53.1442) (-73.5232, -53.3016) (-73.6126, -53.4595) (-73.7014, -53.618) (-73.7895, -53.7772) (-73.8769, -53.9368) (-73.9637, -54.097) (-74.0498, -54.2578) (-74.1352, -54.4191) (-74.22, -54.581) (-74.3042, -54.7434) (-74.3877, -54.9063) (-74.4706, -55.0698) (-74.5528, -55.2337) (-74.6344, -55.3982) (-74.7154, -55.5632) (-74.7958, -55.7287) (-74.8755, -55.8946) (-74.9545, -56.0611) (-75.033, -56.228) (-75.1108, -56.3954) (-75.1881, -56.5633) (-75.2493, -56.698) (-75.295, -56.7993) (-75.3253, -56.8669) (-75.3405, -56.9007) knots 0 0 0 0 0 0 0.01428571 0.02857143 0.04285714 0.05714286 0.07142857 0.08571429 0.1 0.11428571 0.12857143 0.14285714 0.15714286 0.17142857 0.18571429 0.2 0.21428571 0.22857143 0.24285714 0.25714286 0.27142857 0.28571429 0.3 0.31428571 0.32857143 0.34285714 0.35714286 0.37142857 0.38571429 0.4 0.41428571 0.42857143 0.44285714 0.45714286 0.47142857 0.48571429 0.5 0.51428571 0.52857143 0.54285714 0.55714286 0.57142857 0.58571429 0.6 0.61428571 0.62857143 0.64285714 0.65714286 0.67142857 0.68571429 0.7 0.71428571 0.72857143 0.74285714 0.75714286 0.77142857 0.78571429 0.8 0.81428571 0.82857143 0.84285714 0.85714286 0.87142857 0.88571429 0.9 0.91428571 0.92857143 0.94285714 0.95714286 0.97142857 0.98571429 1 1 1 1 1 1
  arc A10 (-75.3405, -56.9007) -> (-72.4465, -60.5296) centre (0.5538, 0.6546) ccw
  spline S3 degree 5 poles (-60.8996, -55.9332) (-60.925, -55.9567) (-60.9765, -56.003) (-61.0553, -56.0704) (-61.1634, -56.1566) (-61.3027, -56.2594) (-61.4449, -56.3586) (-61.5889, -56.4555) (-61.7339, -56.5513) (-61.8796, -56.6462) (-62.0259, -56.7402) (-62.1731, -56.8331) (-62.3215, -56.9245) (-62.4713, -57.014) (-62.6224, -57.1018) (-62.7747, -57.1878) (-62.9282, -57.2725) (-63.0824, -57.3559) (-63.2375, -57.4383) (-63.3932, -57.5197) (-63.5496, -57.6001) (-63.7067, -57.6795) (-63.8646, -57.7577) (-64.0233, -57.8347) (-64.1828, -57.9107) (-64.343, -57.9855) (-64.5039, -58.0593) (-64.6655, -58.1321) (-64.8276, -58.204) (-64.9904, -58.2749) (-65.1538, -58.3449) (-65.3177, -58.4139) (-65.4823, -58.4821) (-65.6474, -58.5492) (-65.8131, -58.6155) (-65.9794, -58.6808) (-66.1462, -58.7453) (-66.3135, -58.8088) (-66.4814, -58.8715) (-66.6498, -58.9334) (-66.8186, -58.9944) (-66.988, -59.0545) (-67.1579, -59.1138) (-67.3282, -59.1723) (-67.499, -59.2299) (-67.6703, -59.2868) (-67.842, -59.3428) (-68.0141, -59.398) (-68.1868, -59.4524) (-68.3598, -59.506) (-68.5333, -59.5588) (-68.7072, -59.6108) (-68.8815, -59.662) (-69.0562, -59.7125) (-69.2313, -59.7622) (-69.4068, -59.8112) (-69.5827, -59.8593) (-69.759, -59.9067) (-69.9357, -59.9534) (-70.1127, -59.9993) (-70.2902, -60.0445) (-70.468, -60.0889) (-70.6461, -60.1326) (-70.8246, -60.1756) (-71.0035, -60.2178) (-71.1827, -60.2593) (-71.3622, -60.3001) (-71.5421, -60.3402) (-71.7223, -60.3795) (-71.9029, -60.4181) (-72.0837, -60.4561) (-72.2287, -60.4858) (-72.3375, -60.5078) (-72.4102, -60.5224) (-72.4465, -60.5296) knots 0 0 0 0 0 0 0.01428571 0.02857143 0.04285714 0.05714286 0.07142857 0.08571429 0.1 0.11428571 0.12857143 0.14285714 0.15714286 0.17142857 0.18571429 0.2 0.21428571 0.22857143 0.24285714 0.25714286 0.27142857 0.28571429 0.3 0.31428571 0.32857143 0.34285714 0.35714286 0.37142857 0.38571429 0.4 0.41428571 0.42857143 0.44285714 0.45714286 0.47142857 0.48571429 0.5 0.51428571 0.52857143 0.54285714 0.55714286 0.57142857 0.58571429 0.6 0.61428571 0.62857143 0.64285714 0.65714286 0.67142857 0.68571429 0.7 0.71428571 0.72857143 0.74285714 0.75714286 0.77142857 0.78571429 0.8 0.81428571 0.82857143 0.84285714 0.85714286 0.87142857 0.88571429 0.9 0.91428571 0.92857143 0.94285714 0.95714286 0.97142857 0.98571429 1 1 1 1 1 1
  line L3 (-60.8996, -55.9332) -> (-59.8002, -54.9212)
  arc A11 (-58.6839, -54.9619) -> (-59.8002, -54.9212) centre (-59.2626, -55.5052) ccw
  arc A12 (-58.6839, -54.9619) -> (-55.0627, -58.5831) centre (0.5538, 0.6546) ccw
  arc A13 (-55.022, -59.6994) -> (-55.0627, -58.5831) centre (-55.606, -59.1618) ccw
  line L4 (-55.022, -59.6994) -> (-56.034, -60.7988)
  spline S4 degree 5 poles (-56.034, -60.7988) (-56.0575, -60.8242) (-56.1038, -60.8757) (-56.1712, -60.9545) (-56.2574, -61.0626) (-56.3602, -61.2019) (-56.4594, -61.3441) (-56.5563, -61.4881) (-56.6521, -61.6331) (-56.747, -61.7788) (-56.841, -61.9251) (-56.9339, -62.0723) (-57.0253, -62.2207) (-57.1148, -62.3705) (-57.2026, -62.5216) (-57.2886, -62.6739) (-57.3733, -62.8274) (-57.4567, -62.9817) (-57.5391, -63.1367) (-57.6205, -63.2924) (-57.7009, -63.4488) (-57.7803, -63.6059) (-57.8585, -63.7638) (-57.9355, -63.9225) (-58.0115, -64.082) (-58.0863, -64.2422) (-58.1601, -64.4031) (-58.2329, -64.5647) (-58.3048, -64.7268) (-58.3757, -64.8896) (-58.4457, -65.053) (-58.5147, -65.2169) (-58.5829, -65.3815) (-58.65, -65.5466) (-58.7163, -65.7123) (-58.7816, -65.8786) (-58.8461, -66.0454) (-58.9096, -66.2127) (-58.9723, -66.3806) (-59.0342, -66.549) (-59.0952, -66.7178) (-59.1553, -66.8872) (-59.2146, -67.0571) (-59.2731, -67.2274) (-59.3307, -67.3982) (-59.3876, -67.5695) (-59.4436, -67.7412) (-59.4988, -67.9133) (-59.5532, -68.086) (-59.6068, -68.259) (-59.6596, -68.4325) (-59.7116, -68.6064) (-59.7628, -68.7807) (-59.8133, -68.9554) (-59.863, -69.1305) (-59.912, -69.306) (-59.9601, -69.4819) (-60.0075, -69.6582) (-60.0542, -69.8349) (-60.1001, -70.0119) (-60.1453, -70.1894) (-60.1897, -70.3672) (-60.2334, -70.5453) (-60.2764, -70.7238) (-60.3186, -70.9027) (-60.3601, -71.0819) (-60.4009, -71.2614) (-60.441, -71.4413) (-60.4803, -71.6215) (-60.5189, -71.8021) (-60.5569, -71.9829) (-60.5866, -72.1279) (-60.6086, -72.2367) (-60.6232, -72.3094) (-60.6304, -72.3457) knots 0 0 0 0 0 0 0.01428571 0.02857143 0.04285714 0.05714286 0.07142857 0.08571429 0.1 0.11428571 0.12857143 0.14285714 0.15714286 0.17142857 0.18571429 0.2 0.21428571 0.22857143 0.24285714 0.25714286 0.27142857 0.28571429 0.3 0.31428571 0.32857143 0.34285714 0.35714286 0.37142857 0.38571429 0.4 0.41428571 0.42857143 0.44285714 0.45714286 0.47142857 0.48571429 0.5 0.51428571 0.52857143 0.54285714 0.55714286 0.57142857 0.58571429 0.6 0.61428571 0.62857143 0.64285714 0.65714286 0.67142857 0.68571429 0.7 0.71428571 0.72857143 0.74285714 0.75714286 0.77142857 0.78571429 0.8 0.81428571 0.82857143 0.84285714 0.85714286 0.87142857 0.88571429 0.9 0.91428571 0.92857143 0.94285714 0.95714286 0.97142857 0.98571429 1 1 1 1 1 1
  arc A14 (-60.6304, -72.3457) -> (-57.0015, -75.2397) centre (0.5538, 0.6546) ccw
  spline S5 degree 5 poles (-46.7668, -68.1891) (-46.7864, -68.2177) (-46.8263, -68.2742) (-46.8882, -68.3575) (-46.9744, -68.4657) (-47.0872, -68.5968) (-47.2038, -68.7252) (-47.3227, -68.8517) (-47.4428, -68.9773) (-47.5636, -69.1023) (-47.6854, -69.2265) (-47.8082, -69.3498) (-47.9325, -69.4719) (-48.0586, -69.5925) (-48.1864, -69.7117) (-48.3158, -69.8295) (-48.4465, -69.9462) (-48.5784, -70.0619) (-48.7112, -70.1767) (-48.8449, -70.2907) (-48.9795, -70.4039) (-49.115, -70.5162) (-49.2516, -70.6276) (-49.3891, -70.7381) (-49.5277, -70.8476) (-49.6672, -70.9562) (-49.8077, -71.0639) (-49.949, -71.1709) (-50.0911, -71.277) (-50.234, -71.3824) (-50.3777, -71.487) (-50.5222, -71.5908) (-50.6674, -71.6938) (-50.8135, -71.796) (-50.9603, -71.8975) (-51.1079, -71.9982) (-51.2562, -72.0981) (-51.4052, -72.1974) (-51.5549, -72.2958) (-51.7053, -72.3936) (-51.8563, -72.4906) (-52.0081, -72.587) (-52.1604, -72.6826) (-52.3135, -72.7775) (-52.4672, -72.8717) (-52.6215, -72.9652) (-52.7765, -73.058) (-52.932, -73.1501) (-53.0882, -73.2416) (-53.245, -73.3323) (-53.4024, -73.4224) (-53.5603, -73.5118) (-53.7188, -73.6006) (-53.878, -73.6887) (-54.0376, -73.7761) (-54.1978, -73.8629) (-54.3586, -73.949) (-54.5199, -74.0344) (-54.6818, -74.1192) (-54.8442, -74.2034) (-55.0071, -74.2869) (-55.1706, -74.3698) (-55.3345, -74.452) (-55.499, -74.5336) (-55.664, -74.6146) (-55.8295, -74.695) (-55.9954, -74.7747) (-56.1619, -74.8537) (-56.3288, -74.9322) (-56.4962, -75.01) (-56.6641, -75.0873) (-56.7988, -75.1485) (-56.9001, -75.1942) (-56.9677, -75.2245) (-57.0015, -75.2397) knots 0 0 0 0 0 0 0.01428571 0.02857143 0.04285714 0.05714286 0.07142857 0.08571429 0.1 0.11428571 0.12857143 0.14285714 0.15714286 0.17142857 0.18571429 0.2 0.21428571 0.22857143 0.24285714 0.25714286 0.27142857 0.28571429 0.3 0.31428571 0.32857143 0.34285714 0.35714286 0.37142857 0.38571429 0.4 0.41428571 0.42857143 0.44285714 0.45714286 0.47142857 0.48571429 0.5 0.51428571 0.52857143 0.54285714 0.55714286 0.57142857 0.58571429 0.6 0.61428571 0.62857143 0.64285714 0.65714286 0.67142857 0.68571429 0.7 0.71428571 0.72857143 0.74285714 0.75714286 0.77142857 0.78571429 0.8 0.81428571 0.82857143 0.84285714 0.85714286 0.87142857 0.88571429 0.9 0.91428571 0.92857143 0.94285714 0.95714286 0.97142857 0.98571429 1 1 1 1 1 1
  line L5 (-46.7668, -68.1891) -> (-45.9202, -66.9578)
  arc A15 (-44.8229, -66.7491) -> (-45.9202, -66.9578) centre (-45.2661, -67.4076) ccw
  arc A16 (-44.8229, -66.7491) -> (-40.4866, -69.4737) centre (0.5538, 0.6546) ccw
  arc A17 (-40.1986, -70.553) -> (-40.4866, -69.4737) centre (-40.8875, -70.1588) ccw
  line L6 (-40.1986, -70.553) -> (-40.9406, -71.85)
  spline S6 degree 5 poles (-40.9406, -71.85) (-40.9578, -71.88) (-40.9914, -71.9405) (-41.0397, -72.0324) (-41.0997, -72.157) (-41.1689, -72.3156) (-41.2339, -72.4763) (-41.2964, -72.6383) (-41.3574, -72.801) (-41.4176, -72.9641) (-41.4767, -73.1277) (-41.5345, -73.2919) (-41.5906, -73.4569) (-41.6445, -73.6228) (-41.6965, -73.7896) (-41.7465, -73.9573) (-41.7949, -74.1257) (-41.8419, -74.2947) (-41.8877, -74.4642) (-41.9324, -74.6341) (-41.976, -74.8045) (-42.0184, -74.9753) (-42.0595, -75.1467) (-42.0993, -75.3185) (-42.1379, -75.4909) (-42.1752, -75.6638) (-42.2113, -75.8371) (-42.2464, -76.0108) (-42.2803, -76.1848) (-42.3133, -76.3593) (-42.3451, -76.5342) (-42.376, -76.7094) (-42.4058, -76.885) (-42.4345, -77.0609) (-42.4622, -77.2372) (-42.4889, -77.4138) (-42.5146, -77.5908) (-42.5394, -77.7681) (-42.5631, -77.9457) (-42.586, -78.1236) (-42.6079, -78.3018) (-42.6288, -78.4803) (-42.6488, -78.6591) (-42.6679, -78.8382) (-42.6861, -79.0175) (-42.7034, -79.1971) (-42.7198, -79.377) (-42.7353, -79.5572) (-42.7499, -79.7375) (-42.7637, -79.9182) (-42.7766, -80.0991) (-42.7886, -80.2802) (-42.7998, -80.4615) (-42.8101, -80.6431) (-42.8196, -80.8249) (-42.8282, -81.0069) (-42.8361, -81.1891) (-42.8431, -81.3715) (-42.8492, -81.5541) (-42.8546, -81.737) (-42.8592, -81.92) (-42.8629, -82.1032) (-42.8659, -82.2866) (-42.868, -82.4702) (-42.8694, -82.654) (-42.87, -82.8379) (-42.8698, -83.022) (-42.8688, -83.2063) (-42.8671, -83.3908) (-42.8646, -83.5754) (-42.8613, -83.7602) (-42.8581, -83.9081) (-42.8553, -84.0191) (-42.8533, -84.0932) (-42.8523, -84.1302) knots 0 0 0 0 0 0 0.01428571 0.02857143 0.04285714 0.05714286 0.07142857 0.08571429 0.1 0.11428571 0.12857143 0.14285714 0.15714286 0.17142857 0.18571429 0.2 0.21428571 0.22857143 0.24285714 0.25714286 0.27142857 0.28571429 0.3 0.31428571 0.32857143 0.34285714 0.35714286 0.37142857 0.38571429 0.4 0.41428571 0.42857143 0.44285714 0.45714286 0.47142857 0.48571429 0.5 0.51428571 0.52857143 0.54285714 0.55714286 0.57142857 0.58571429 0.6 0.61428571 0.62857143 0.64285714 0.65714286 0.67142857 0.68571429 0.7 0.71428571 0.72857143 0.74285714 0.75714286 0.77142857 0.78571429 0.8 0.81428571 0.82857143 0.84285714 0.85714286 0.87142857 0.88571429 0.9 0.91428571 0.92857143 0.94285714 0.95714286 0.97142857 0.98571429 1 1 1 1 1 1
  arc A18 (-42.8523, -84.1302) -> (-38.6704, -86.1441) centre (0.5538, 0.6546) ccw
  spline S7 degree 5 poles (-30.2612, -76.9929) (-30.274, -77.0251) (-30.3003, -77.0891) (-30.342, -77.1841) (-30.402, -77.3087) (-30.4829, -77.4617) (-30.568, -77.6127) (-30.6557, -77.7626) (-30.7448, -77.9118) (-30.8349, -78.0605) (-30.9259, -78.2087) (-31.0182, -78.3563) (-31.1123, -78.5029) (-31.2083, -78.6486) (-31.3064, -78.7932) (-31.4063, -78.9369) (-31.5078, -79.0797) (-31.6106, -79.2218) (-31.7145, -79.3633) (-31.8195, -79.5042) (-31.9255, -79.6445) (-32.0327, -79.7842) (-32.141, -79.9232) (-32.2506, -80.0615) (-32.3613, -80.1991) (-32.4732, -80.336) (-32.5861, -80.4723) (-32.7001, -80.608) (-32.815, -80.7431) (-32.9309, -80.8776) (-33.0477, -81.0116) (-33.1655, -81.1449) (-33.2842, -81.2777) (-33.4038, -81.4098) (-33.5244, -81.5414) (-33.6458, -81.6724) (-33.7682, -81.8029) (-33.8914, -81.9328) (-34.0154, -82.0621) (-34.1403, -82.1909) (-34.2659, -82.3191) (-34.3924, -82.4468) (-34.5197, -82.5739) (-34.6478, -82.7005) (-34.7767, -82.8265) (-34.9063, -82.952) (-35.0368, -83.077) (-35.1679, -83.2014) (-35.2998, -83.3253) (-35.4325, -83.4487) (-35.5659, -83.5715) (-35.7, -83.6939) (-35.8348, -83.8157) (-35.9703, -83.9369) (-36.1065, -84.0577) (-36.2434, -84.178) (-36.381, -84.2977) (-36.5193, -84.4169) (-36.6582, -84.5356) (-36.7978, -84.6538) (-36.938, -84.7715) (-37.0789, -84.8886) (-37.2205, -85.0053) (-37.3627, -85.1214) (-37.5055, -85.2371) (-37.649, -85.3522) (-37.793, -85.4669) (-37.9377, -85.581) (-38.083, -85.6947) (-38.2289, -85.8078) (-38.3754, -85.9205) (-38.4931, -86.0102) (-38.5816, -86.0772) (-38.6408, -86.1218) (-38.6704, -86.1441) knots 0 0 0 0 0 0 0.01428571 0.02857143 0.04285714 0.05714286 0.07142857 0.08571429 0.1 0.11428571 0.12857143 0.14285714 0.15714286 0.17142857 0.18571429 0.2 0.21428571 0.22857143 0.24285714 0.25714286 0.27142857 0.28571429 0.3 0.31428571 0.32857143 0.34285714 0.35714286 0.37142857 0.38571429 0.4 0.41428571 0.42857143 0.44285714 0.45714286 0.47142857 0.48571429 0.5 0.51428571 0.52857143 0.54285714 0.55714286 0.57142857 0.58571429 0.6 0.61428571 0.62857143 0.64285714 0.65714286 0.67142857 0.68571429 0.7 0.71428571 0.72857143 0.74285714 0.75714286 0.77142857 0.78571429 0.8 0.81428571 0.82857143 0.84285714 0.85714286 0.87142857 0.88571429 0.9 0.91428571 0.92857143 0.94285714 0.95714286 0.97142857 0.98571429 1 1 1 1 1 1
  line L7 (-30.2612, -76.9929) -> (-29.7098, -75.6041)
  arc A19 (-28.6864, -75.1564) -> (-29.7098, -75.6041) centre (-28.9721, -75.897) ccw
  arc A20 (-28.6864, -75.1564) -> (-23.8526, -76.8478) centre (0.5538, 0.6546) ccw
  arc A21 (-23.3316, -77.8359) -> (-23.8526, -76.8478) centre (-24.091, -77.6049) ccw
  line L8 (-23.3316, -77.8359) -> (-23.7664, -79.2655)